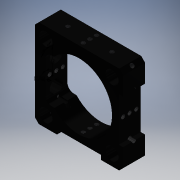
# Autodesk Inventor part: G061042000
Saved by Autodesk Inventor 2017 (Build 210142000, 142)
## iProperties
Part Number: G061042000
Material: Generisch
Document SubType Name: Modeling
Designer: David Merges
Density: 1 g/cm^3
Appearance: Eloxiert - schwarz
Author: David Merges
Autodesk Inventor part; units mm, degrees
note: some values were not read from the file. Chosen so that the rebuilt part matches the saved one: direction of "Bohrung4".
ref_plane "YZ Plane" through (0, 0, 0) normal (1, 0, 0) x (0, 1, 0)
ref_plane "XZ Plane" through (0, 0, 0) normal (0, 1, 0) x (-1, 0, 0)
ref_plane "XY Plane" through (0, 0, 0) normal (0, 0, 1) x (1, 0, 0)
sketch "Skizze1" plane through (0, 0, 0) normal (0, 1, 0) x (-1, 0, 0)
  line L0 (20, 20) -> (-20, 20)
  line L1 (-20, 20) -> (-20, -20)
  line L2 (-20, -20) -> (20, -20)
  line L3 (20, -20) -> (20, 20)
  line L4 (20, -20) -> (-20, 20) construction
  point P0 (0, 0)
  point P1 (0, 0)
  dimension "d0" = 40
  dimension "d1" = 40
  constraints: 10 end point, 2 parallel, 1 coincident, 1 horizontal, 1 midpoint, 1 perpendicular
  measures "d0" distance of L2.end L1.end
  measures "d1" distance of L1.end L0.end
extrude "Extrusion1" add sketch "Skizze1" along normal mid plane 10
sketch "Skizze2" plane through (0, -5, 0) normal (0, -1, 0) x (1, 0, 0)
  line L0 (-15, 15) -> (15, 15) construction
  line L1 (15, 15) -> (15, -15) construction
  line L2 (15, -15) -> (-15, -15) construction
  line L3 (-15, -15) -> (-15, 15) construction
  line L4 (15, -15) -> (-15, 15) construction
  point P0 (0, 0)
  dimension "d4" = 30
  dimension "d5" = 30
  constraints: 10 end point, 2 midpoint, 2 parallel, 1 horizontal, 1 perpendicular
  measures "d4" distance of L1.end L2.end
  measures "d5" distance of L0.end L1.end
hole "Bohrung1" at (15, -5, -15) at (15, -5, 15) at (-15, -5, 15) at (-15, -5, -15) direction (0, 1, 0) diameter 6 end through all
sketch "Skizze3" plane through (0, -5, 0) normal (0, -1, 0) x (1, 0, 0)
  circle A0 centre (-15, 15) radius 3 projected
  circle A1 centre (15, -15) radius 3 projected
  circle A2 centre (15, 15) radius 3 projected
  circle A3 centre (-15, -15) radius 3 projected
  line L0 (20, 20) -> (-20, 20) projected
  line L1 (-20, 20) -> (-20, -20) projected
  line L2 (-20, -20) -> (20, -20) projected
  line L3 (20, -20) -> (20, 20) projected
  line L4 (-20, 18.2322) -> (-18.2322, 20)
  line L5 (-20, 20) -> (20, 20) projected
  line L6 (20, 20) -> (-20, 20) projected
  line L7 (-18.2322, 20) -> (-20, 20)
  line L8 (-20, 20) -> (-20, 18.2322)
  point P0 (0, 0)
  dimension "d13" = 45
  dimension "d14" = 2.5
  constraints: 6 end point, 2 collinear, 2 point on line
  measures "d13" angle of L0 L4
  measures "d14" distance of L4.start L4.end
extrude "Extrusion2" cut sketch "Skizze3" against normal through all contours L4 L1 L0
pattern_circular "Runde Anordnung1" count 4 over 360 about axis through (0, -10, 0) along (0, 1, 0) of "Extrusion2"
sketch "Skizze8" plane through (20, -5, -18.2322) normal (1, 0, 0) x (0, 0, -1)
  line L0 (-36.4645, 10) -> (-36.4645, 0) projected
  line L1 (0, 0) -> (0, 10) projected
  line L2 (-28.2322, 5) -> (-8.2322, 5) construction
  line L3 (-36.4645, 0) -> (-36.4645, 10) construction
  line L4 (-36.4645, 0) -> (0, 10) construction
  point P0 (-18.2322, 5)
  dimension "d37" = 20
  constraints: 4 end point, 2 coincident, 2 midpoint, 1 perpendicular
  measures "d37" distance of L2.start L2.end
hole "Bohrung3" at (20, 0, 10) at (20, 0, -10) direction (-1, 0, 0) diameter 1.813 depth 10 tip angle 118 thread size "M2.3x0.45" class "6H" standard "ISO Metric profile"
pattern_circular "Runde Anordnung2" count 4 over 360 about axis through (0, -10, 0) along (0, 1, 0) of "Bohrung3"
sketch "Skizze9" plane through (18.2322, -5, 20) normal (0.7071068, 0, 0.7071068) x (0.7071068, 0, -0.7071068)
  line L0 (2.5, 0) -> (0, 0) projected
  line L1 (0, 10) -> (2.5, 10) projected
  line L2 (2.5, 10) -> (2.5, 0) construction
  line L3 (0, 10) -> (0, 0) construction
  line L4 (2.5, 0) -> (0, 10) construction
  point P0 (1.25, 5)
  point P1 (1.25, 5)
  constraints: 2 end point, 1 coincident
hole "Bohrung4" at (19.1161, 0, 19.1161) direction (-0.7071068, 0, -0.7071068) diameter 1.813 end up to surface thread size "M2.3x0.45" class "6H" standard "ISO Metric profile"
pattern_circular "Runde Anordnung3" count 4 over 360 about axis through (0, -10, 0) along (0, 1, 0) of "Bohrung4"
sketch "Skizze10" plane through (0, -5, 0) normal (0, -1, 0) x (1, 0, 0)
  circle A0 centre (0, 0) radius 15
  dimension "d58" = 30
  constraints: 1 centre point, 1 coincident
  measures "d58" diameter of A0
extrude "Extrusion6" cut sketch "Skizze10" against normal through all
sketch "Skizze11" plane through (-18.2322, -5, 20) normal (0, 0, 1) x (1, 0, 0)
  line L0 (3.2322, 10) -> (33.2322, 10) construction
  line L1 (18.2322, 10) -> (18.2322, 0) construction
  line L2 (33.2322, 0) -> (3.2322, 0) construction
  point P0 (18.2322, 5)
  point P1 (18.2322, 5)
  point P2 (18.2322, 5)
  point P3 (18.2322, 8)
  point P4 (18.2322, 2)
  dimension "d61" = 2
  dimension "d62" = 2
  constraints: 2 coincident, 2 end point, 2 midpoint, 2 point on line
  measures "d61" distance of point (18.232, 8) L1.start
  measures "d62" distance from line of L2 point (18.232, 2)
hole "Bohrung5" at (0, 0, 20) at (0, 3, 20) at (0, -3, 20) direction (0, 0, -1) diameter 1.813 depth 7.2 tip angle 118 thread size "M2.3x0.45" class "6H" standard "ISO Metric profile"
pattern_circular "Runde Anordnung4" count 4 over 360 about axis through (0, -10, 0) along (0, 1, 0) of "Bohrung5"
sketch "Skizze12" plane through (-18.2322, -5, 20) normal (0, 0, 1) x (1, 0, 0)
  line L0 (24.2322, 5) -> (12.2322, 5) construction
  point P0 (18.2322, 5)
  point P1 (18.2322, 5)
  dimension "d73" = 12
  constraints: 2 end point, 1 coincident, 1 horizontal, 1 midpoint
  measures "d73" distance of L0.start L0.end
sketch "Skizze13" plane through (20, -5, -18.2322) normal (1, 0, 0) x (0, 0, -1)
  line L0 (-28.2322, 0) -> (-8.2322, 0)
  line L1 (-8.2322, 0) -> (-8.2322, 10)
  line L2 (-8.2322, 10) -> (-28.2322, 10)
  line L3 (-28.2322, 10) -> (-28.2322, 0)
  line L4 (-28.2322, 0) -> (-8.2322, 10) construction
  point P0 (-18.2322, 5)
  point P1 (-18.2322, 5)
  dimension "d92" = 20
  dimension "d93" = 10
  constraints: 10 end point, 2 parallel, 1 coincident, 1 horizontal, 1 midpoint, 1 perpendicular
  measures "d92" distance of L2.end L1.end
  measures "d93" distance of L1.end L0.end
extrude "Extrusion7" cut sketch "Skizze13" against normal blind 2
sketch "Skizze14" plane through (18.2322, 5, -20) normal (0, 0, -1) x (-1, 0, 0)
  line L0 (8.2322, -10) -> (28.2322, -10)
  line L1 (28.2322, -10) -> (28.2322, 0)
  line L2 (28.2322, 0) -> (8.2322, 0)
  line L3 (8.2322, 0) -> (8.2322, -10)
  line L4 (8.2322, -10) -> (28.2322, 0) construction
  point P0 (18.2322, -5)
  point P1 (18.2322, -5)
  dimension "d96" = 20
  dimension "d97" = 10
  constraints: 10 end point, 2 parallel, 1 coincident, 1 horizontal, 1 midpoint, 1 perpendicular
  measures "d96" distance of L2.end L1.end
  measures "d97" distance of L1.end L0.end
extrude "Extrusion8" cut sketch "Skizze14" against normal blind 2
sketch "Skizze16" plane through (0, -5, 0) normal (0, -1, 0) x (1, 0, 0)
  line L0 (-20, 0) -> (-15.3, 0) construction
  line L1 (-12.3, 9.9041) -> (-5.3, 9.9041)
  line L2 (-5.3, 9.9041) -> (-5.3, -10.0959)
  line L3 (-5.3, -10.0959) -> (-12.3, -10.0959)
  line L4 (-15.3, -7.0959) -> (-15.3, 6.9041)
  arc A0 (-12.3, 9.9041) -> (-15.3, 6.9041) centre (-12.3, 6.9041) ccw
  arc A1 (-15.3, -7.0959) -> (-12.3, -10.0959) centre (-12.3, -7.0959) ccw
  line L5 (-20, 18.2322) -> (-20, -18.2322) projected
  point P0 (0, 0)
  point P1 (-15.3, -10.0959)
  dimension "d112" = 4.7
  dimension "d113" = 10
  dimension "d114" = 20
  dimension "d115" = 3
  dimension "d116" = 3
  constraints: 10 end point, 4 point on circle, 4 tangent, 3 point on line, 2 centre point, 2 horizontal, 2 parallel, 1 midpoint, 1 perpendicular
  measures "d112" distance of L0.start L0.end
  measures "d113" distance of L2.end point (-15.3, -10.096)
  measures "d114" distance of L1.end L2.end
  measures "d115" radius of A0
  measures "d116" radius of A1
extrude "Extrusion9" cut sketch "Skizze16" against normal blind 10
sketch "Skizze17" plane through (-20, -5, 18.2322) normal (-1, 0, 0) x (0, 0, 1)
  line L0 (-24.2322, 5) -> (-12.2322, 5) construction
  line L1 (-24.2322, 5) -> (-12.2322, 5) construction
  circle A0 centre (-12.2322, 5) radius 3
  circle A1 centre (-12.2322, 5) radius 2
  circle A2 centre (-24.2322, 5) radius 2
  circle A3 centre (-24.2322, 5) radius 3
  point P0 (-18.2322, 5)
  point P1 (-18.2322, 5)
  dimension "d119" = 12
  dimension "d120" = 0
  dimension "d121" = 6
  dimension "d122" = 4
  dimension "d123" = 4
  dimension "d124" = 6
  constraints: 7 coincident, 4 centre point, 4 end point, 2 horizontal, 1 collinear, 1 midpoint
  measures "d119" distance of L0.start L0.end
  measures "d120" distance between parallel lines of L0 L1
  measures "d121" diameter of A0
  measures "d122" diameter of A1
  measures "d123" diameter of A2
  measures "d124" diameter of A3
extrude "Extrusion10" cut sketch "Skizze17" against normal blind 5 contours A0 | A1 | A2 | A3
equation "\"d115\" = d116"
